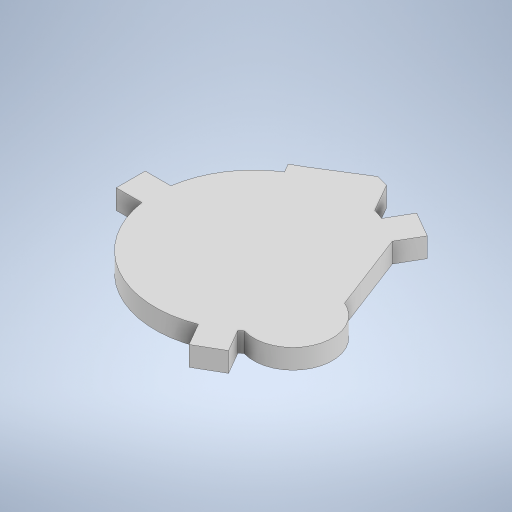
# Autodesk Inventor part: Electronic base
Saved by Autodesk Inventor 2024 (Build 280153000, 153)
## iProperties
Created: 2024-03-27
Part Number: Electronic base
Material: Generic
Document SubType Name: Modeling
Designer: auror
Density: 1 g/cm^3
Appearance: Default
Author: auror
Autodesk Inventor part; units mm, degrees
ref_plane "YZ Plane" through (0, 0, 0) normal (1, 0, 0) x (0, 1, 0)
ref_plane "XZ Plane" through (0, 0, 0) normal (0, 1, 0) x (-1, 0, 0)
ref_plane "XY Plane" through (0, 0, 0) normal (0, 0, 1) x (1, 0, 0)
sketch "Sketch9" plane through (0, 0, 0) normal (0, 1, 0) x (-1, 0, 0)
  line L0 (37.6236, 0) -> (-39.3749, 0) construction
  line L1 (0, 0) -> (-26.8726, 46.5447) construction
  line L2 (0, 0) -> (-26.275, -45.5096) construction
  line L3 (31.2294, 3.6686) -> (31.2294, -3.6686)
  line L4 (31.2294, 3.6686) -> (24.7294, 3.6686)
  line L5 (31.2294, -3.6686) -> (24.7294, -3.6686)
  line L6 (0, 0) -> (-18.4784, 42.9064) construction
  line L7 (0, 0) -> (-25.1787, 33.7798) construction
  line L8 (0, 0) -> (31.2294, 3.6686) construction
  line L9 (-12.4376, 28.8797) -> (-18.7918, 25.2111)
  line L10 (-12.4376, 28.8797) -> (-9.1876, 23.2506)
  line L11 (-18.7918, 25.2111) -> (-15.5418, 19.582)
  line L12 (0, 0) -> (-18.2948, -42.48) construction
  line L13 (-18.2948, -42.48) -> (0, 0) construction
  line L14 (0, 0) -> (-26.6993, -35.8199) construction
  line L15 (-18.7918, -25.2111) -> (-12.4376, -28.8797)
  line L16 (-18.7918, -25.2111) -> (-15.5418, -19.582)
  line L17 (-12.4376, -28.8797) -> (-9.1876, -23.2506)
  arc A0 (-15.5418, 19.582) -> (-15.5418, -19.582) centre (0, 0) ccw
  arc A1 (-9.1876, -23.2506) -> (24.7294, -3.6686) centre (0, 0) ccw
  arc A2 (24.7294, 3.6686) -> (-9.1876, 23.2506) centre (0, 0) ccw
  line L18 (0, 0) -> (31.2294, -3.6686) construction
  dimension "d131" = 120
  dimension "d132" = 120
  dimension "d136" = 6.7
  dimension "d137" = 6.7
  dimension "d139" = 6.7
  dimension "d140" = 6.7
  dimension "d220" = 6.5
  dimension "d221" = 6.5
  dimension "d222" = 25
  dimension "d223" = 25
  dimension "d224" = 25
  dimension "d225" = 6.5
  dimension "d227" = 6.5
  dimension "d228" = 6.5
  dimension "d236" = 6.7
  dimension "d237" = 6.7
  constraints: 38 end point, 6 point on circle, 4 perpendicular, 4 point on line, 3 centre point, 3 horizontal, 2 coincident, 1 vertical
  measures "d131" angle of L2 L0
  measures "d132" angle of L1 L0
  measures "d136" angle of L1 L6
  measures "d137" angle of L7 L1
  measures "d139" angle of L2 L12
  measures "d140" angle of L2 L14
  measures "d220" distance of L15.end L17.end
  measures "d221" distance of L9.end L11.end
  measures "d222" radius of A0
  measures "d223" radius of A1
  measures "d224" radius of A2
  measures "d225" distance of L3.end L5.end
  measures "d227" distance of L9.start L10.end
  measures "d228" distance of L15.start L16.end
  measures "d236" angle of L0 L8
  measures "d237" angle of L18 L0
extrude "Extrusion4" add sketch "Sketch9" along normal blind 5
sketch "Sketch17" plane through (0, 5, 0) normal (0, 1, 0) x (1, 0, 0)
  arc A0 (15.5418, -19.582) -> (15.5418, 19.582) centre (0, 0) ccw projected
  line L0 (15.5418, 19.582) -> (24.6527, -4.1527)
  arc A1 (24.6527, -4.1527) -> (15.5418, 19.582) centre (0, 0) ccw
  line L1 (39.1744, 0) -> (-46.6954, 0) construction
  dimension "d244" = 69
  constraints: 4 end point, 3 point on circle, 1 centre point, 1 coincident, 1 horizontal
  measures "d244" angle of L1 L0
extrude "Extrusion8" cut sketch "Sketch17" against normal through all
sketch "Sketch38" plane through (0, 5, 0) normal (0, 1, 0) x (1, 0, 0)
  line L0 (2.4652, 31.2084) -> (-0.476, 31.9965) projected
  line L1 (-0.476, 31.9965) -> (-11.5905, 25.0753)
  line L2 (8.3534, 21.0097) -> (2.4652, 31.2084) projected
  line L3 (-0.476, 31.9965) -> (2.4652, 31.2084)
  arc A0 (9.1876, 23.2506) -> (-24.7294, 3.6686) centre (0, 0) ccw projected
  line L4 (2.4652, 31.2084) -> (6.5546, 24.1255)
  arc A1 (6.2227, 24.2132) -> (14.6024, -20.2921) centre (0, 0) ccw
  line L5 (-11.0461, 17.1324) -> (-13.356, 21.1333) projected
  line L6 (-13.356, 21.1333) -> (-14.6216, 23.3253)
  line L7 (-14.6216, 23.3253) -> (-11.5905, 25.0753)
  line L8 (-13.356, 21.1333) -> (-6.4888, 10.7302)
  line L9 (-6.4888, 10.7302) -> (6.2227, 24.2132)
  point P0 (3.9242, 24.6901)
  point P1 (8.9539, -17.5087)
  point P2 (6.5546, 24.1255)
  constraints: 14 end point, 2 point on circle, 1 centre point, 1 coincident, 1 collinear, 1 perpendicular
extrude "Extrusion24" add sketch "Sketch38" against normal blind 5 contours L2 A0 L6 L7 L1 L0
sketch "Sketch43" plane through (0, 5, 0) normal (0, 1, 0) x (1, 0, 0)
  circle A0 centre (19.2133, -9.2784) radius 10
  arc A1 (12.0096, -16.2143) -> (26.417, -2.3425) centre (19.2133, -9.2784) ccw projected
  point P0 (0, 0)
  dimension "d385" = 20
  constraints: 1 centre point, 1 concentric
  measures "d385" diameter of A0
extrude "Extrusion28" add sketch "Sketch43" against normal blind 5
body "Solid2"
